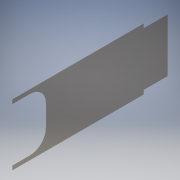
# Autodesk Inventor part: Giant PC Plate
Saved by Autodesk Inventor 2019.4 (Build 234330000, 330)
## iProperties
Created: 2020-01-10
Part Number: Giant PC Plate
Material: Polycarbonate, Smoke
Document SubType Name: Modeling
Designer: Mark
Mass: 357.956 g
Surface Area: 5996.34 cm^2
Volume: 298.297 cm^3
Density: 1.2 g/cm^3
Appearance: Polycarbonate - Smoked
Author: Mark
Autodesk Inventor part; units mm, degrees
ref_plane "YZ Plane" through (0, 0, 0) normal (1, 0, 0) x (0, 1, 0)
ref_plane "XZ Plane" through (0, 0, 0) normal (0, 1, 0) x (-1, 0, 0)
ref_plane "XY Plane" through (0, 0, 0) normal (0, 0, 1) x (1, 0, 0)
sketch "Sketch1" plane through (0, 0, 0) normal (1, 0, 0) x (0, 1, 0)
  line L0 (-191.5, 485) -> (191.5, 485)
  line L1 (191.5, 485) -> (191.5, -485)
  line L2 (191.5, -485) -> (-191.5, -485)
  line L3 (-191.5, -485) -> (-191.5, 485)
  line L4 (-191.5, 485) -> (191.5, -485) construction
  line L5 (191.5, 485) -> (-191.5, -485) construction
  point P0 (0, 0)
  dimension "d0" = 383
  dimension "d1" = 970
  constraints: 12 end point, 2 midpoint, 2 parallel, 1 horizontal, 1 perpendicular
  measures "d0" distance of L1.end L2.end
  measures "d1" distance of L0.end L1.end
extrude "Extrusion1" add sketch "Sketch1" along normal blind 1
sketch "Sketch2" plane through (1, 0, 0) normal (1, 0, 0) x (0, 0, -1)
  line L0 (-485, 191.5) -> (-485, -191.5) projected
  line L1 (-485, 166.5) -> (-275, 166.5)
  line L2 (-275, 166.5) -> (-275, -166.5)
  line L3 (-275, -166.5) -> (-485, -166.5)
  line L4 (-485, -166.5) -> (-485, 166.5)
  line L5 (485, 191.5) -> (-485, 191.5) projected
  line L6 (335, 166) -> (485, 166)
  line L7 (485, 166) -> (485, -166.5) construction
  line L8 (485, -166.5) -> (335, -166.5)
  line L9 (335, -166.5) -> (335, 166) construction
  line L10 (335, 166) -> (485, -166.5) construction
  line L11 (485, 166) -> (335, -166.5) construction
  line L12 (485, -191.5) -> (485, 191.5) projected
  line L13 (-485, -191.5) -> (485, -191.5) projected
  line L14 (335, 166) -> (485, 166)
  line L15 (485, 166) -> (485, 191.5)
  line L16 (485, 191.5) -> (335, 191.5)
  line L17 (335, 191.5) -> (335, 166)
  line L18 (335, -166.5) -> (485, -166.5)
  line L19 (485, -166.5) -> (485, -191.5)
  line L20 (485, -191.5) -> (335, -191.5)
  line L21 (335, -191.5) -> (335, -166.5)
  point P0 (0, 0)
  point P1 (410, -0.25)
  dimension "d4" = 210
  dimension "d5" = 333
  dimension "d12" = 25
  dimension "d13" = 150
  dimension "d14" = 332.5
  dimension "d15" = 25
  constraints: 36 end point, 8 parallel, 4 horizontal, 4 perpendicular, 2 midpoint, 1 collinear, 1 point on line
  measures "d4" distance of L2.end L3.end
  measures "d5" distance of L1.end L2.end
  measures "d12" distance between parallel lines of L5 L1
  measures "d13" distance of L7.end L8.end
  measures "d14" distance of L6.end L7.end
  measures "d15" distance between parallel lines of L13 L8
extrude "Extrusion2" cut sketch "Sketch2" against normal blind 1 contours L1 L2 L3 L0 | L5 L12 L6 L17 | L21 L8 L12 L13
fillet "Fillet1" radius 100 2 edges at (0.5, 166.5, 275) (0.5, -166.5, 275)
body "Solid1"
